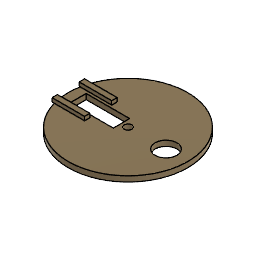
pot lid v3 (Autodesk Fusion 360 design; units mm, degrees)
Autodesk Fusion 360 part; units mm, degrees
cylinder "CylinderPrimitive1" add diameter 110 height 5 placed x (1, 0, 0) y (0, 1, 0) z (0, 0, 1) at (0, 0, 0)
sketch "Sketch3" plane through (0, 0, 5) normal (0, 0, 1) x (-1, 0, 0)
  circle A0 centre (0, 0) radius 55
  circle A1 centre (0, 0) radius 3.5
  line L0 (46, -7.5) -> (6, -7.5)
  line L1 (6, -7.5) -> (6, 7.5)
  line L2 (6, 7.5) -> (46, 7.5)
  line L3 (46, 7.5) -> (46, -7.5)
  line L4 (55, 10) -> (25, 10)
  line L5 (25, 10) -> (25, 15)
  line L6 (25, 15) -> (55, 15)
  line L7 (55, 15) -> (55, 10)
  line L8 (55, -15) -> (25, -15)
  line L9 (25, -15) -> (25, -10)
  line L10 (25, -10) -> (55, -10)
  line L11 (55, -10) -> (55, -15)
  circle A2 centre (-35, 0) radius 10
  dimension "d3" = 7
  dimension "d4" = 40
  dimension "d5" = 15
  dimension "d6" = 7.5
  dimension "d7" = 6
  dimension "d8" = 20
  dimension "d9" = 25
  dimension "d10" = 25
  dimension "d11" = 10
  dimension "d12" = 5
  dimension "d13" = 5
  dimension "d14" = 30
  dimension "d15" = 30
  dimension "d16" = 35
  dimension "d17" = 20
  constraint coincident A0.centre A1.centre
  constraint horizontal L0
  constraint vertical L1
  constraint horizontal L2
  constraint vertical L3
  constraint horizontal L4
  constraint vertical L5
  constraint horizontal L6
  constraint vertical L7
  constraint horizontal L8
  constraint vertical L9
  constraint horizontal L10
  constraint vertical L11
  measures "d3" diameter of A1
  measures "d4" distance of L1.end L2.end
  measures "d5" distance of L0.start L2.end
  measures "d6" vertical distance of A0.centre L1.end
  measures "d7" distance of A0.centre L1
  measures "d8" distance of L4 L10
  measures "d9" distance of A0.centre L9
  measures "d10" horizontal distance of A0.centre L4.end
  measures "d11" vertical distance of A0.centre L4.end
  measures "d12" distance of L8.end L9.end
  measures "d13" distance of L4.end L5.end
  measures "d14" distance of L8.start L8.end
  measures "d15" distance of L5.end L6.end
  measures "d16" distance of A0.centre A2.centre
  measures "d17" diameter of A2
extrude "Extrude1" cut sketch "Sketch3" against normal through all contours A1 | L0 L1 L2 L3 | A2
extrude "Extrude2" add sketch "Sketch3" along normal blind 3.5 contours A0 L4 L5 L6 | A0 L4 L6 L7 | A0 L8 L10 L11 | A0 L8 L9 L10
